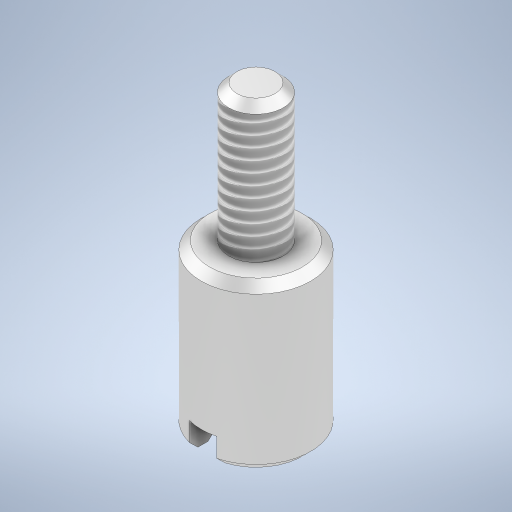
# Autodesk Inventor part: BRU-2006S
Saved by Autodesk Inventor 2024.2 (Build 282272000, 272)
## iProperties
Created: 2024-01-03
Part Number: BRU-2006S
Material: Stainless Steel AISI 304
Document SubType Name: Modeling
Designer: Masato Kubotera
Density: 8 g/cm^3
Appearance: Chrome - Satin
Catalog Web Link: https://www.hirosugi-net.co.jp/shop/g/g8454/
Vendor: HIROSUGI
Author: Masato Kubotera
Autodesk Inventor part; units mm, degrees
ref_plane "YZ Plane" through (0, 0, 0) normal (1, 0, 0) x (0, 1, 0)
ref_plane "XZ Plane" through (0, 0, 0) normal (0, 1, 0) x (-1, 0, 0)
ref_plane "XY Plane" through (0, 0, 0) normal (0, 0, 1) x (1, 0, 0)
sketch "Sketch1" plane through (0, 0, 0) normal (0, 1, 0) x (-1, 0, 0)
  line L0 (0, 0) -> (-2, 0)
  line L1 (-2, 0) -> (-2, 6)
  line L2 (-2, 6) -> (-1, 6)
  line L3 (-1, 6) -> (-1, 11)
  line L4 (-1, 11) -> (0, 11)
  line L5 (0, 11) -> (0, 0)
  dimension "d1" = 5
  dimension "d2" = 6
  dimension "d3" = 2
  dimension "d4" = 4
  constraints: 12 end point, 3 horizontal, 2 vertical, 1 perpendicular
  measures "d1" distance of L2.end L3.end
  measures "d2" distance of L0.end L1.end
  measures "d3" diameter of L3 L5
  measures "d4" diameter of L1 L5
revolve "Revolution1" add sketch "Sketch1" angle 360 about axis through (0, 0, 11) along (0, 0, -1)
sketch "Sketch2" plane through (0, 0, 0) normal (0, 0, -1) x (-1, 0, 0)
  line L0 (-2, -0.5) -> (2, -0.5)
  line L1 (2, -0.5) -> (2, 0.5)
  line L2 (2, 0.5) -> (-2, 0.5)
  line L3 (-2, 0.5) -> (-2, -0.5)
  line L4 (-2, -0.5) -> (2, 0.5) construction
  line L5 (2, -0.5) -> (-2, 0.5) construction
  circle A0 centre (0, 0) radius 2 projected
  dimension "d6" = 1
  constraints: 12 end point, 2 midpoint, 2 parallel, 1 horizontal, 1 perpendicular, 1 tangent
  measures "d6" distance of L1.end L0.end
extrude "Extrusion1" cut sketch "Sketch2" against normal blind 1 contours L3 A0 L0 | A0 L2 L0 | L3 L2 A0 | A0 L1 L0 | A0 L2 L1
hole "Hole1" at (0, 0, 0) direction (0, 0, 1) diameter 2.1129 depth 5 thread size "M2.6x0.45" class "6H" standard "ANSI Metric M Profile"
thread "Thread1" size "M2x0.4" class "6g" standard "ANSI Metric M Profile" full length
chamfer "Chamfer1" distance 0.3 angle 45 7 edges at (-2, 0, 6) (0, 2, 0) (0, -2, 0) (0, -1.0564, 0) (-0.5421, 0.9067, 0) (0.5421, 0.9067, 0) (-1, 0, 11)
body "Solid1"
